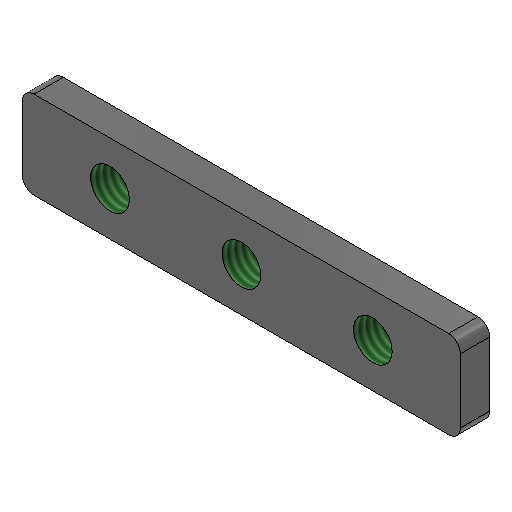
# Autodesk Inventor part: TL20240701-10100CV-005
Saved by Autodesk Inventor 2022.5 (Build 265521000, 521)
## iProperties
Category: CONVEYOR ASSY
Company: 현대 트랜시스(대유)
Created: 2023-04-10
Part Number: TL20240701-10100CV-005
Checked By: 김형민
Engr Approved By: 김시현
User Status: 116
Material: SS400
Description: 0
Document SubType Name: Modeling
Mfg Approved By: 호상태
Designer: 박성규
Stock Number: 005
Density: 7.85 g/cm^3
Appearance: Plating Zinc White
Project: SW PJT
DETAIL: Coveryor Assembly
M/C TITLE: CJ 제일제당 협동로봇 포장시스탬 PILOT 장비
PARTS NAME: Bracket
SPECIFICATION: TA20221101-CV200000-015
DocNumber: 221118_Standard_v1
Folder: .\
VDS_Category: 엔지니어링
Detail Description: Processed products
Title: NUT PLATE
Subject: SW차종 시트조립라인
Author: 박성규
Revision Number: A
Autodesk Inventor part; units mm, degrees
ref_plane "YZ Plane" through (0, 0, 0) normal (1, 0, 0) x (0, 1, 0)
ref_plane "XZ Plane" through (0, 0, 0) normal (0, 1, 0) x (-1, 0, 0)
ref_plane "XY Plane" through (0, 0, 0) normal (0, 0, 1) x (1, 0, 0)
sketch "스케치9" plane through (0, 0, 0) normal (0, 0, 1) x (1, 0, 0)
  line L0 (-37.5, -7.5) -> (37.5, -7.5)
  line L1 (37.5, -7.5) -> (37.5, 7.5)
  line L2 (37.5, 7.5) -> (-37.5, 7.5)
  line L3 (-37.5, 7.5) -> (-37.5, -7.5)
  line L4 (-37.5, -7.5) -> (37.5, 7.5) construction
  line L5 (37.5, -7.5) -> (-37.5, 7.5) construction
  point P0 (0, 0)
  dimension "d40" = 75
  dimension "d41" = 15
  constraints: 12 end point, 2 midpoint, 2 parallel, 1 horizontal, 1 perpendicular
  measures "d40" distance of L1.end L2.end
  measures "d41" distance of L0.end L1.end
extrude "돌출4" add sketch "스케치9" along normal blind 5
fillet "모깎기2" radius 2 4 edges at (37.5, 7.5, 2.5) (37.5, -7.5, 2.5) (-37.5, 7.5, 2.5) (-37.5, -7.5, 2.5)
sketch "스케치10" plane through (0, 0, 5) normal (0, 0, 1) x (1, 0, 0)
  point P0 (0, 0)
  point P1 (0, 0)
  point P2 (-22.5, 0)
  point P3 (22.5, 0)
  dimension "d45" = 22.5
  dimension "d46" = 22.5
  constraints: 2 horizontal alignment, 1 coincident
  measures "d45" distance of point (0, 0) point (22.5, 0)
  measures "d46" distance of point (-22.5, 0) point (0, 0)
hole "구멍3" at (0, 0, 5) at (-22.5, 0, 5) at (22.5, 0, 5) direction (0, 0, -1) diameter 6.647 end through all thread size "M8x1.25" class "6H" standard "TS profile"
equation "\"d46\" = d45"
